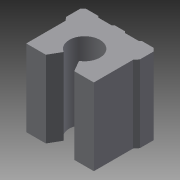
# Autodesk Inventor part: sbr20uu
Saved by Autodesk Inventor 2014 (Build 180170000, 170)
## iProperties
Created: 2014-10-05
Part Number: sbr20uu
Material: Generic
Document SubType Name: Modeling
Designer: Matthew
Density: 1 g/cm^3
Appearance: Default
Author: Matthew
Autodesk Inventor part; units mm, degrees
ref_plane "YZ Plane" through (0, 0, 0) normal (1, 0, 0) x (0, 1, 0)
ref_plane "XZ Plane" through (0, 0, 0) normal (0, 1, 0) x (-1, 0, 0)
sketch "Sketch2" plane through (0, 0, 0) normal (0, 0, 1) x (1, 0, 0)
  arc A0 (5, -12.1603) -> (-5, -12.1603) centre (0, -3.5) ccw
  line L0 (-5, -12.1603) -> (5, -12.1603) construction
  line L1 (5, -12.1603) -> (9.2376, -19.5)
  line L2 (-5, -12.1603) -> (-9.2376, -19.5)
  line L3 (-24, 8.5) -> (-22, 6.0385)
  line L4 (-22, 6.0385) -> (-22, -19.5)
  line L5 (24, 8.5) -> (22, 6.0385)
  line L6 (-22, -19.5) -> (-9.2376, -19.5)
  line L7 (22, 6.0385) -> (22, -19.5)
  line L8 (22, -19.5) -> (9.2376, -19.5)
  line L9 (-24, 17.5) -> (-22, 19.5)
  line L10 (-24, 17.5) -> (-24, 8.5)
  line L11 (24, 8.5) -> (24, 17.5)
  line L12 (24, 17.5) -> (22, 19.5)
  line L13 (-22, 19.5) -> (-14.125, 19.5)
  line L14 (-14.125, 19.5) -> (-13.125, 18.5)
  line L15 (-13.125, 18.5) -> (-4.375, 18.5)
  line L16 (-4.375, 18.5) -> (-3.375, 19.5)
  line L17 (-3.375, 19.5) -> (3.375, 19.5)
  line L18 (3.375, 19.5) -> (4.375, 18.5)
  line L19 (4.375, 18.5) -> (13.125, 18.5)
  line L20 (13.125, 18.5) -> (14.125, 19.5)
  line L21 (14.125, 19.5) -> (22, 19.5)
  point P0 (0, 0)
  point P1 (0, 0)
  point P2 (0, 0)
  dimension "h1" = 10
  dimension "r1" = 10
  dimension "d15" = 2
  dimension "d16" = 2
  dimension "d18" = 25.5385
  dimension "d19" = 25.5385
  dimension "d20" = 12.7624
  dimension "d21" = 12.7624
  dimension "d22" = 7.3398
  dimension "d23" = 7.3398
  dimension "d24" = 2.4615
  dimension "d25" = 2.4615
  dimension "d26" = 3.5
  dimension "d27" = 18.4752
  dimension "d28" = 22
  dimension "d33" = 2
  dimension "d34" = 2
  dimension "d35" = 9
  dimension "d36" = 2
  dimension "d37" = 44
  dimension "d38" = 9
  dimension "d40" = 1
  dimension "d41" = 8.75
  dimension "d42" = 8.75
  dimension "d43" = 6.75
  dimension "d44" = 1
  dimension "d45" = 1
  dimension "d46" = 1
  dimension "d47" = 7.875
  dimension "d48" = 7.875
  constraints: 44 end point, 8 perpendicular, 5 parallel, 2 coincident, 2 point on circle, 1 centre point, 1 vertical alignment
  measures "h1" distance of L0.start L0.end
  measures "r1" radius of A0
  measures "d15" horizontal distance of L3.start L3.end
  measures "d16" horizontal distance of L5.start L5.end
  measures "d18" distance of L3.end L4.end
  measures "d19" distance of L5.end L7.end
  measures "d20" distance of L7.end L1.end
  measures "d21" distance of L4.end L2.end
  measures "d22" vertical distance of L0.start L2.end
  measures "d23" vertical distance of L0.end L1.end
  measures "d24" vertical distance of L5.start L5.end
  measures "d25" vertical distance of L3.start L3.end
  measures "d26" distance of A0.centre point (0, 0)
  measures "d27" distance of L1.end L2.end
  measures "d28" distance from line of L7 A0.centre
  measures "d33" horizontal distance of L9.start L9.end
  measures "d34" horizontal distance of L9.start L9.end
  measures "d35" distance of L5.start L11.end
  measures "d36" horizontal distance of L11.end L12.end
  measures "d37" distance of L9.end L12.end
  measures "d38" distance of L9.start L3.start
  measures "d40" horizontal distance of L13.end L14.end
  measures "d41" distance of L14.end L15.end
  measures "d42" distance of L18.end L19.end
  measures "d43" distance of L16.end L17.end
  measures "d44" horizontal distance of L15.end L16.end
  measures "d45" horizontal distance of L17.end L18.end
  measures "d46" horizontal distance of L19.end L20.end
  measures "d47" distance of L20.end L12.end
  measures "d48" distance of L9.end L13.end
extrude "Extrusion1" add sketch "Sketch2" along normal blind 50
ref_plane "Work Plane1" through (-3.375, 19.5, 0) normal (0, 1, 0) x (1, 0, 0)
sketch "Sketch3" plane through (-3.375, 19.5, 0) normal (0, 1, 0) x (1, 0, 0)
  line L0 (-20.625, 0) -> (3.375, 0) construction
  line L1 (-20.625, 0) -> (-20.625, -15.5497) construction
  line L2 (27.375, 0) -> (27.375, -50) construction
  line L3 (-18.625, 0) -> (-18.625, -50) construction
  line L4 (25.375, 0) -> (25.375, -50) construction
  point P0 (-14.125, -7.5)
  point P1 (20.875, -7.5)
  point P2 (-14.125, -42.5)
  point P3 (20.875, -42.5)
  dimension "d52" = 35
  dimension "d55" = 35
  dimension "d58" = 7.5
  dimension "d68" = 2
  dimension "d69" = 4.5
  dimension "d70" = 2
  dimension "d71" = 4.5
  constraints: 4 end point, 2 horizontal, 1 perpendicular, 1 vertical, 3 other
  measures "d52" distance of point (-14.125, -7.5) point (20.875, -7.5)
  measures "d55" distance of point (-14.125, -7.5) point (-14.125, -42.5)
  measures "d58" distance from line of L0 point (-14.125, -7.5)
  measures "d68" distance between parallel lines of L1 L3
  measures "d69" distance from line of point (-14.125, -7.5) L3
  measures "d70" distance between parallel lines of L2 L4
  measures "d71" distance from line of L4 point (20.875, -7.5)
hole "Hole1" at (-17.5, 19.5, 7.5) at (17.5, 19.5, 7.5) at (-17.5, 19.5, 42.5) at (17.5, 19.5, 42.5) direction (0, -1, 0) diameter 6.3 depth 12 tip angle 118
equation "\"d16\" = d15"
equation "\"d19\" = d18"
equation "\"d21\" = d20"
equation "\"d23\" = d22"
equation "\"d25\" = d24"
equation "\"d34\" = d33"
equation "\"d42\" = d41"
equation "\"d44\" = d40"
equation "\"d45\" = d40"
equation "\"d46\" = d40"
equation "\"d48\" = d47"
body "Solid1"
